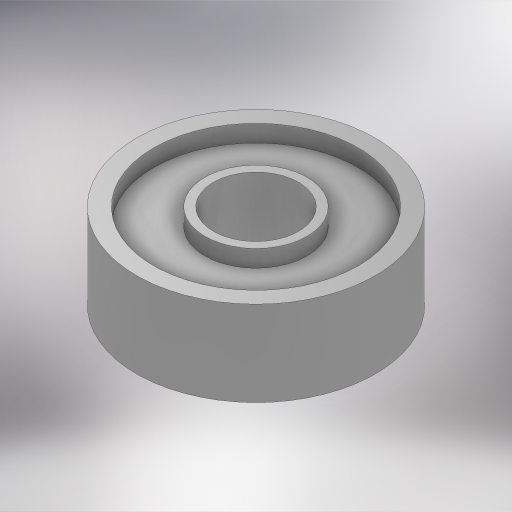
# Autodesk Inventor part: Bearing5X15X5
Saved by Autodesk Inventor 2024.3 (Build 283343000, 343)
## iProperties
Created: 2025-03-28
Part Number: Bearing5X15X5
Material: Generic
Document SubType Name: Modeling
Designer: danie
Density: 1 g/cm^3
Appearance: Default
Author: danie
Autodesk Inventor part; units mm, degrees
ref_plane "YZ Plane" through (0, 0, 0) normal (1, 0, 0) x (0, 1, 0)
ref_plane "XZ Plane" through (0, 0, 0) normal (0, 1, 0) x (-1, 0, 0)
sketch "Sketch1" plane through (0, 0, 0) normal (0, 1, 0) x (-1, 0, 0)
  circle A0 centre (0, 0) radius 7
  circle A1 centre (0, 0) radius 2.5
  dimension "d0" = 14
  dimension "d1" = 5
  constraints: 2 centre point, 2 coincident
  measures "d0" diameter of A0
  measures "d1" diameter of A1
extrude "Extrusion1" add sketch "Sketch1" along normal blind 5
sketch "Sketch2" plane through (0, 5, 0) normal (0, 1, 0) x (1, 0, 0)
  circle A0 centre (0, 0) radius 7 projected
  circle A1 centre (0, 0) radius 2.5 projected
  circle A2 centre (0, 0) radius 3
  circle A3 centre (0, 0) radius 6
  dimension "d4" = 6
  dimension "d5" = 1
  constraints: 2 centre point, 2 coincident
  measures "d4" diameter of A2
  measures "d5" radial gap between concentric circles of A3 A0
extrude "Extrusion2" cut sketch "Sketch2" against normal blind 1 contours A3
ref_plane "Work Plane1" through (0, 2.5, 0) normal (0, 1, 0) x (1, 0, 0)
mirror "Mirror1" about plane through (0, 2.5, 0) normal (0, 1, 0) of "Extrusion2"
body "Solid1"
